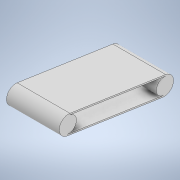
# Autodesk Inventor part: ShootingMech_Housing4
Saved by Autodesk Inventor 2020 (Build 240168000, 168)
## iProperties
Created: 2022-01-22
Part Number: ShootingMech_Housing4
Material: Generic
Document SubType Name: Modeling
Designer: danie
Density: 1 g/cm^3
Appearance: Default
Author: danie
Autodesk Inventor part; units mm, degrees
ref_plane "YZ Plane" through (0, 0, 0) normal (1, 0, 0) x (0, 1, 0)
ref_plane "XZ Plane" through (0, 0, 0) normal (0, 1, 0) x (-1, 0, 0)
ref_plane "XY Plane" through (0, 0, 0) normal (0, 0, 1) x (1, 0, 0)
sketch "Sketch3" plane through (0, 0, 0) normal (1, 0, 0) x (0, 1, 0)
  line L0 (17.2137, 115.1798) -> (-17.2137, -115.1798) construction
  line L1 (-4.7671, 118.4649) -> (-39.1946, -111.8947)
  line L2 (4.7671, -118.4649) -> (39.1946, 111.8947)
  arc A0 (39.1946, 111.8947) -> (-4.7671, 118.4649) centre (17.2137, 115.1798) ccw
  arc A1 (-39.1946, -111.8947) -> (4.7671, -118.4649) centre (-17.2137, -115.1798) ccw
  line L3 (0, 0) -> (232.918, 0) construction
  line L4 (36.0545, 112.364) -> (1.627, -117.9956)
  arc A2 (-36.0545, -112.364) -> (1.627, -117.9956) centre (-17.2137, -115.1798) ccw
  line L5 (-36.0545, -112.364) -> (-1.627, 117.9956)
  arc A3 (36.0545, 112.364) -> (-1.627, 117.9956) centre (17.2137, 115.1798) ccw
  ellipse E0 centre (17.2137, 115.1798) end of major axis (36.0545, 112.364) minor radius 19.05
  ellipse E1 centre (-17.2137, -115.1798) end of major axis (1.627, -117.9956) minor radius 19.05
  point P0 (-36.0545, -112.364)
  dimension "d8" = 116.459
  dimension "d9" = 98.5
  dimension "d10" = 44.45
  dimension "d11" = 3.175
  constraints: 14 end point, 8 point on circle, 4 centre point, 4 tangent, 2 coincident, 2 parallel, 1 equal length, 1 horizontal, 1 midpoint, 11 other
  measures "d8" distance of L3.start L0.end
  measures "d9" angle of L0 L3
  measures "d10" diameter of A1
  measures "d11" distance between parallel lines of L2 L4
extrude "Extrusion3" add sketch "Sketch3" along normal blind 127 contours A0 L2 A1 L1 | E0 A3 | A2 E1
body "Solid2"
